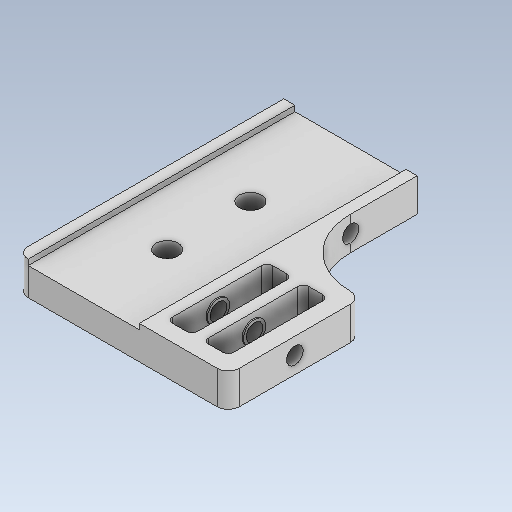
# Autodesk Inventor part: leftshortNEW
Saved by Autodesk Inventor 2020 (Build 240168000, 168)
## iProperties
Created: 2019-12-18
Part Number: leftshortNEW
Material: Generic
Document SubType Name: Modeling
Designer: xj82b
Density: 1 g/cm^3
Appearance: Default
Author: xj82b
Autodesk Inventor part; units mm, degrees
ref_plane "YZ Plane" through (0, 0, 0) normal (1, 0, 0) x (0, 1, 0)
ref_plane "XZ Plane" through (0, 0, 0) normal (0, 1, 0) x (-1, 0, 0)
ref_plane "XY Plane" through (0, 0, 0) normal (0, 0, 1) x (1, 0, 0)
sketch "Sketch6" plane through (0, 0, 0) normal (0, 1, 0) x (-1, 0, 0)
  line L0 (0, 0) -> (-24, 0)
  line L1 (-24, 0) -> (-24, -48)
  line L2 (-24, -48) -> (0, -48)
  line L3 (0, -48) -> (0, 0)
  line L4 (-24, -24) -> (-38, -24)
  line L5 (-38, -24) -> (-38, 0)
  line L6 (-38, 0) -> (-24, 0)
  line L7 (-24, 0) -> (-24, -24)
  line L8 (-24, -21) -> (-35, -21)
  line L9 (-35, -21) -> (-35, -3)
  line L10 (-35, -3) -> (-24, -3)
  line L11 (-24, -3) -> (-24, -21)
  circle A0 centre (-12, -15) radius 2
  circle A1 centre (-12, -30) radius 2
  line L12 (-28.5, -21) -> (-30.5, -21)
  line L13 (-30.5, -21) -> (-30.5, -3)
  line L14 (-30.5, -3) -> (-28.5, -3)
  line L15 (-28.5, -3) -> (-28.5, -21)
  point P0 (-12, 0)
  dimension "d35" = 24
  dimension "d36" = 48
  dimension "d37" = 14
  dimension "d38" = 24
  dimension "d39" = 3
  dimension "d40" = 3
  dimension "d41" = 3
  dimension "d42" = 4
  dimension "d43" = 4
  dimension "d44" = 15
  dimension "d45" = 30
  dimension "d46" = 4.5
  dimension "d47" = 4.5
  constraints: 32 end point, 8 parallel, 4 horizontal, 4 perpendicular, 3 point on line, 2 centre point, 2 midpoint, 2 vertical alignment
  measures "d35" distance of L2.end L1.end
  measures "d36" distance of L0.end L1.end
  measures "d37" distance of L5.end L6.end
  measures "d38" distance of L4.end L5.end
  measures "d39" distance between parallel lines of L4 L8
  measures "d40" distance between parallel lines of L5 L9
  measures "d41" distance between parallel lines of L6 L10
  measures "d42" diameter of A0
  measures "d43" diameter of A1
  measures "d44" distance from line of A0.centre L0
  measures "d45" distance from line of A1.centre L0
  measures "d46" distance between parallel lines of L11 L15
  measures "d47" distance between parallel lines of L9 L13
extrude "Extrusion6" add sketch "Sketch6" along normal blind 6 contours L3 L2 L1 L0 | L1 L10 L9 L8 L4 L5 L6 | L15 L8 L13 L10
sketch "Sketch7" plane through (0, 6, 0) normal (0, 1, 0) x (1, 0, 0)
  line L0 (2, 50.5567) -> (22, 50.5567)
  line L1 (22, 50.5567) -> (22, -3.9772)
  line L2 (22, -3.9772) -> (2, -3.9772)
  line L3 (2, -3.9772) -> (2, 50.5567)
  line L4 (0, 48) -> (0, 0) projected
  dimension "d50" = 2
  dimension "d51" = 20
  constraints: 8 end point, 2 parallel, 1 horizontal, 1 perpendicular
  measures "d50" distance between parallel lines of L4 L3
  measures "d51" distance between parallel lines of L1 L3
extrude "Extrusion7" cut sketch "Sketch7" against normal blind 1
sketch "Sketch8" plane through (38, 0, 0) normal (1, 0, 0) x (0, 0, -1)
  circle A0 centre (12, 3) radius 1.5
  line L0 (0, 6) -> (24, 6) projected
  line L1 (24, 0) -> (24, 6) projected
  point P0 (0, 0)
  point P1 (12, 6)
  point P2 (24, 3)
  dimension "d54" = 3
  constraints: 2 midpoint, 1 centre point, 1 horizontal alignment, 1 vertical alignment
  measures "d54" diameter of A0
extrude "Extrusion8" cut sketch "Sketch8" against normal through all
sketch "Sketch9" plane through (24, 0, -3) normal (1, 0, 0) x (0, 0, -1)
  circle A0 centre (9, 3) radius 1.5
  circle A1 centre (9, 3) radius 1.5 projected
  circle A2 centre (9, 3) radius 2
  point P0 (-3, 0)
  dimension "d57" = 3
  dimension "d58" = 4
  constraints: 2 centre point, 2 concentric
  measures "d57" diameter of A0
  measures "d58" diameter of A2
extrude "Extrusion9" add sketch "Sketch9" along normal blind 12
sketch "Sketch10" plane through (0, 6, 0) normal (0, 1, 0) x (1, 0, 0)
  line L0 (30.75, 19.1618) -> (34.75, 19.1618)
  line L1 (34.75, 19.1618) -> (34.75, 4.3826)
  line L2 (34.75, 4.3826) -> (30.75, 4.3826)
  line L3 (30.75, 4.3826) -> (30.75, 19.1618)
  line L4 (24.25, 18.4541) -> (28.25, 18.4541)
  line L5 (28.25, 18.4541) -> (28.25, 6.1312)
  line L6 (28.25, 6.1312) -> (24.25, 6.1312)
  line L7 (24.25, 6.1312) -> (24.25, 18.4541)
  line L8 (30.5, 3) -> (30.5, 21) projected
  line L9 (24, 3) -> (24, 21) projected
  point P0 (0, 0)
  dimension "d61" = 4
  dimension "d62" = 4
  dimension "d63" = 0.25
  dimension "d64" = 0.25
  constraints: 16 end point, 4 parallel, 2 horizontal, 2 perpendicular
  measures "d61" distance of L1.end L2.end
  measures "d62" distance of L5.end L6.end
  measures "d63" distance between parallel lines of L8 L3
  measures "d64" distance between parallel lines of L9 L7
extrude "Extrusion10" cut sketch "Sketch10" against normal through all
sketch "Sketch11" plane through (24, 0, -24) normal (1, 0, 0) x (0, 0, -1)
  circle A0 centre (12, 3) radius 1.5
  line L0 (24, 0) -> (24, 6) projected
  point P0 (-24, 0)
  point P1 (24, 3)
  dimension "d67" = 3
  dimension "d68" = 12
  constraints: 1 centre point, 1 horizontal alignment, 1 midpoint
  measures "d67" diameter of A0
  measures "d68" distance from line of L0 A0.centre
extrude "Extrusion11" cut sketch "Sketch11" against normal through all
fillet "Fillet1" radius 12 1 edges at (24, 3, -24)
fillet "Fillet2" radius 2 2 edges at (38, 3, -24) (0, 3, 0)
fillet "Fillet3" radius 1 8 edges at (24, 3, -21) (30.5, 3, -21) (24, 3, -3) (30.5, 3, -3) (35, 3, -21) (28.5, 3, -21) (28.5, 3, -3) (35, 3, -3)
body "Solid2"
